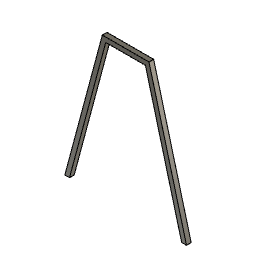
Table chair set v2 (Autodesk Fusion 360 archive; units mm, degrees)
design "Seat leg"
Autodesk Fusion 360 part; units mm, degrees
sketch "Sketch1" plane through (0, 0, 0) normal (0, 1, 0) x (1, 0, 0)
  line L0 (0, -450) -> (-46.5874, -450) construction
  line L1 (0, -450) -> (150, -450)
  line L2 (0, 0) -> (-131.645, 0)
  line L3 (-131.645, 0) -> (-284.4079, 0)
  line L4 (0, -450) -> (-120.5771, 0)
  line L5 (0, -450) -> (-465.8743, -450) construction
  line L6 (150, -450) -> (269.5369, -3.8823)
  line L7 (-120.5771, 0) -> (-105.5771, 0)
  line L8 (-105.5771, 0) -> (10.9808, -435)
  line L9 (-105.5771, 0) -> (345.8241, 0) construction
  line L10 (10.9808, -435) -> (138.4901, -435)
  line L11 (138.4901, -435) -> (255.048, 0)
  line L12 (269.5369, -3.8823) -> (270.5771, 0)
  line L13 (255.048, 0) -> (270.5771, 0)
  dimension "d3" = 150
  dimension "d5" = 75
  dimension "d6" = 75
  dimension "d8" = 15
  dimension "d9" = 75
  dimension "d10" = 75
  dimension "d11" = 15
  dimension "d12" = 15
  dimension "d13" = 15
  constraint horizontal L0
  constraint coincident L2.start origin
  constraint horizontal L5
  constraint coincident L2 L4.end
  constraint parallel L2 L7
  constraint horizontal L9
  constraint coincident L9 L11.end
  constraint coincident L9 L12.end
  constraint parallel L11 L12
  measures "d3" distance of L0.start L1.end
  measures "d5" angle of L4 L5
  measures "d6" angle of L5 L6
  measures "d8" distance of L4.end L7.end
  measures "d9" angle of L8 L9
  measures "d10" angle of L10 L11
  measures "d11" distance of L6 L11
  measures "d12" distance of L1 L10
  measures "d13" distance of L6.end L11.end
extrude "Extrude1" add sketch "Sketch1" along normal blind 15 makes body 1
copy_body "Body->Comp1" bodies 1 removing the originals makes body 2 in component "Seat leg"
component "Seat leg" placed x (1, 0, 0) y (0, 1, 0) z (0, 0, 1) at (0, 0, 0)
